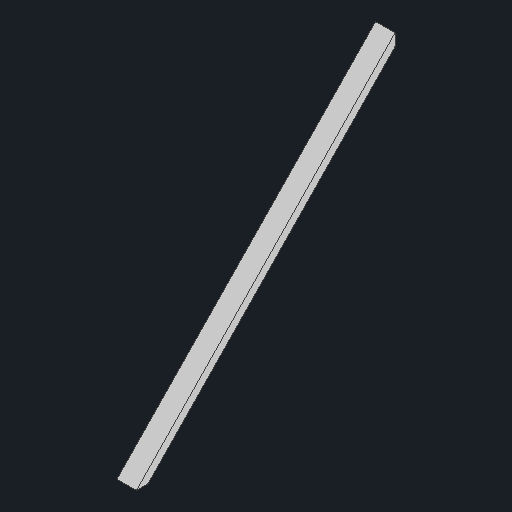
# Autodesk Inventor part: S_2x4x66.83
Saved by Autodesk Inventor 2026 (Build 300175000, 175)
## iProperties
Created: 2025-08-28
Part Number: S_2x4x66.83
Material: Generic
Document SubType Name: Modeling
Designer: trott
Density: 1 g/cm^3
Appearance: Default
Author: trott
Autodesk Inventor part; units mm, degrees
ref_plane "YZ Plane" through (0, 0, 0) normal (1, 0, 0) x (0, 1, 0)
ref_plane "XZ Plane" through (0, 0, 0) normal (0, 1, 0) x (-1, 0, 0)
ref_plane "XY Plane" through (0, 0, 0) normal (0, 0, 1) x (1, 0, 0)
sketch "Sketch1" plane through (0, 0, 0) normal (1, 0, 0) x (0, 1, 0)
  line L0 (-609.6, 590.55) -> (609.6, 590.55)
  line L1 (609.6, 590.55) -> (609.6, -590.55)
  line L2 (609.6, -590.55) -> (-609.6, -590.55)
  line L3 (-609.6, -590.55) -> (-609.6, 590.55)
  line L4 (-609.6, 590.55) -> (609.6, -590.55) construction
  line L5 (609.6, 590.55) -> (-609.6, -590.55) construction
  line L6 (-609.6, 590.55) -> (609.6, -590.55)
  line L7 (0, 0) -> (-27.365, -26.5098)
  line L8 (-609.6, 537.5304) -> (554.8701, -590.55)
  dimension "d0" = 1219.2
  dimension "d1" = 1181.1
  dimension "d2" = 38.1
  constraints: 18 end point, 3 midpoint, 3 parallel, 2 point on line, 1 collinear, 1 horizontal, 1 perpendicular
  measures "d0" distance of L1.end L2.end
  measures "d1" distance of L2.end L0.start
  measures "d2" distance of L7.start L7.end
extrude "Extrusion1" add sketch "Sketch1" along normal blind 88.9 contours L6 L7 L8 L3 | L6 L2 L8 L7
body "Solid1"
